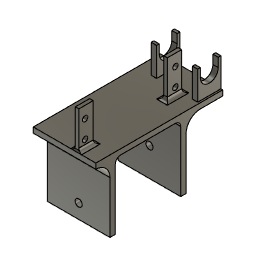
Servo_bracket v13 (Autodesk Fusion 360 design; units mm, degrees)
Autodesk Fusion 360 part; units mm, degrees
sketch "Sketch1" plane through (0, 0, 0) normal (0, 0, 1) x (1, 0, 0)
  line L0 (0, 0) -> (35, 0)
  line L1 (35, 0) -> (35, 71)
  line L2 (35, 71) -> (0, 71)
  line L3 (0, 71) -> (0, 0)
  dimension "d1" = 35
  dimension "d2" = 71
  constraint horizontal L0
  constraint vertical L1
  constraint horizontal L2
  constraint vertical L3
  constraint coincident L0.start L3.end
  measures "d1" distance of L0.start L0.end
  measures "d2" distance of L0.start L2.end
extrude "Extrude1" add sketch "Sketch1" along normal blind 3
sketch "Sketch2" plane through (0, 0, 3) normal (0, 0, 1) x (-1, 0, 0)
  line L0 (0, -71) -> (0, 0)
  line L1 (0, 0) -> (-35, 0)
  line L2 (-35, 0) -> (-35, -71)
  line L3 (-35, -71) -> (0, -71)
  line L4 (-25, -0.5) -> (-23, -0.5)
  line L5 (-23, -0.5) -> (-23, -8.5)
  line L6 (-23, -8.5) -> (-25, -8.5)
  line L7 (-25, -8.5) -> (-25, -0.5)
  line L8 (0, 0) -> (-35, 0)
  line L9 (-25, -58) -> (-23, -58)
  line L10 (-23, -58) -> (-23, -50)
  line L11 (-23, -50) -> (-25, -50)
  line L12 (-25, -50) -> (-25, -58)
  line L13 (-35, 0) -> (-35, -71)
  dimension "d5" = 0.5
  dimension "d6" = 2
  dimension "d7" = 8
  dimension "d8" = 2
  dimension "d9" = 8
  dimension "d10" = 41.5
  dimension "d11" = 10
  dimension "d12" = 10
  constraint horizontal L4
  constraint vertical L5
  constraint horizontal L6
  constraint vertical L7
  constraint horizontal L9
  constraint vertical L10
  constraint horizontal L11
  constraint vertical L12
  measures "d5" distance of L4 L8
  measures "d6" distance of L5.end L6.end
  measures "d7" distance of L4.end L5.end
  measures "d8" distance of L9.start L9.end
  measures "d9" distance of L9.end L10.end
  measures "d10" distance of L6 L11
  measures "d11" distance of L7 L13
  measures "d12" distance of L12 L13
extrude "Extrude2" add sketch "Sketch2" along normal blind 21 contours L4 L5 L6 L7 | L9 L10 L11 L12
sketch "Sketch4" plane through (25, 0, 0) normal (1, 0, 0) x (0, 1, 0)
  line L0 (0.5, 3) -> (8.5, 3)
  line L1 (8.5, 3) -> (8.5, 24)
  line L2 (8.5, 24) -> (0.5, 24)
  line L3 (0.5, 24) -> (0.5, 3)
  circle A0 centre (4, 7.5) radius 1.5
  circle A1 centre (4, 17.5) radius 1.5
  circle A2 centre (54.5, 7.5) radius 1.5
  circle A3 centre (54.5, 17.5) radius 1.5
  line L4 (58, 3) -> (50, 3)
  line L5 (50, 3) -> (50, 24)
  dimension "d15" = 3
  dimension "d16" = 4.5
  dimension "d17" = 3.5
  dimension "d18" = 3
  dimension "d19" = 10
  dimension "d20" = 3.5
  dimension "d21" = 3
  dimension "d22" = 3
  dimension "d23" = 4.5
  dimension "d24" = 4.5
  dimension "d25" = 10
  dimension "d26" = 4.5
  measures "d15" diameter of A0
  measures "d16" distance of L0 A0.centre
  measures "d17" distance of L3 A0.centre
  measures "d18" diameter of A1
  measures "d19" distance of A0.centre A1.centre
  measures "d20" distance of L3 A1.centre
  measures "d21" diameter of A2
  measures "d22" diameter of A3
  measures "d23" distance of A2.centre L4
  measures "d24" distance of A2.centre L5
  measures "d25" distance of A2.centre A3.centre
  measures "d26" distance of A3.centre L5
extrude "Extrude3" cut sketch "Sketch4" against normal up to surface (2 mm away) contours A0 | A1 | A2 | A3
sketch "Sketch5" plane through (0, 0, 3) normal (0, 0, 1) x (-1, 0, 0)
  line L0 (-25, -8.5) -> (-25, -0.5)
  line L1 (-25, -0.5) -> (-23, -0.5)
  line L2 (-23, -0.5) -> (-23, -8.5)
  line L3 (-23, -8.5) -> (-25, -8.5)
  line L4 (-25, -50) -> (-23, -50)
  line L5 (-23, -50) -> (-23, -58)
  line L6 (-23, -58) -> (-25, -58)
  line L7 (-25, -58) -> (-25, -50)
  line L8 (0, -71) -> (0, 0)
  line L9 (0, 0) -> (-35, 0)
  line L10 (-35, 0) -> (-35, -71)
  line L11 (-35, -71) -> (0, -71)
  line L12 (-31, -58) -> (-34, -58)
  line L13 (-34, -58) -> (-34, -71)
  line L14 (-34, -71) -> (-31, -71)
  line L15 (-31, -71) -> (-31, -58)
  line L16 (-8, -58) -> (-11, -58)
  line L17 (-11, -58) -> (-11, -71)
  line L18 (-11, -71) -> (-8, -71)
  line L19 (-8, -71) -> (-8, -58)
  dimension "d30" = 13
  dimension "d31" = 3
  dimension "d32" = 1
  dimension "d33" = 13
  dimension "d34" = 3
  dimension "d37" = 20
  constraint horizontal L12
  constraint vertical L13
  constraint horizontal L14
  constraint vertical L15
  constraint horizontal L16
  constraint vertical L17
  constraint horizontal L18
  constraint vertical L19
  constraint coincident L10.end L14
  constraint coincident L8.start L18
  measures "d30" distance of L12.start L14.end
  measures "d31" distance of L12.start L12.end
  measures "d32" distance of L10 L13
  measures "d33" distance of L16.start L18.end
  measures "d34" distance of L16.start L16.end
  measures "d37" distance of L15 L17
extrude "Extrude4" add sketch "Sketch5" along normal blind 16 contours L11 L16 L17 L18 L19 | L11 L12 L13 L14 L15
sketch "Sketch6" plane through (34, 0, 0) normal (1, 0, 0) x (0, 1, 0)
  line L0 (58, 3) -> (71, 3)
  line L1 (71, 3) -> (71, 19)
  line L2 (71, 19) -> (58, 19)
  line L3 (58, 19) -> (58, 3)
  line L4 (59.5, 14) -> (59.5, 19)
  line L5 (69.5, 14) -> (69.5, 19)
  line L6 (59.5, 19) -> (69.5, 19)
  arc A0 (59.5, 14) -> (69.5, 14) centre (64.5, 14) ccw
  dimension "d40" = 10
  dimension "d42" = 1.5
  dimension "d43" = 11
  constraint coincident L2 L4.end
  constraint tangent L4 A0
  constraint perpendicular L2 L4
  constraint coincident L2 L5.end
  constraint tangent L5 A0
  constraint perpendicular L2 L5
  measures "d40" diameter of A0
  measures "d42" distance of L3 L4
  measures "d43" distance of L0 A0.centre
extrude "Extrude8" cut sketch "Sketch6" against normal up to surface (26 mm away) contours L2 L4 L5 L6 A0
extrude "Extrude5" cut sketch "Sketch6" against normal up to surface (26 mm away) contours L2 L4 L5 L6 A0
fillet "Fillet1" radius 2 3 edges at (25, 4.5, 3) (24, 8.5, 3) (23, 4.5, 3)
fillet "Fillet2" radius 1 1 edges at (24, 0.5, 3)
fillet "Fillet3" radius 2 4 edges at (25, 54, 3) (24, 50, 3) (23, 54, 3) (24, 58, 3)
sketch "Sketch8" plane through (0, 0, 3) normal (0, 0, 1) x (-1, 0, 0)
  line L0 (-31, -71) -> (-11, -71)
  line L1 (-34, -71) -> (-34, -58)
  line L2 (-34, -58) -> (-31, -58)
  line L3 (-31, -58) -> (-31, -71)
  line L4 (-8, -71) -> (0, -71)
  line L5 (-11, -71) -> (-11, -58)
  line L6 (-11, -58) -> (-8, -58)
  line L7 (-8, -58) -> (-8, -71)
  line L8 (-21, 0) -> (-21, -10.5)
  line L9 (-21, -10.5) -> (-27, -10.5)
  line L10 (-27, -10.5) -> (-27, 0)
  line L11 (-27, 0) -> (-35, 0)
  line L12 (-35, 0) -> (-35, -71)
  line L13 (-35, -71) -> (-34, -71)
  line L14 (0, -71) -> (0, 0)
  line L15 (0, 0) -> (-21, 0)
  line L16 (-21, -60) -> (-27, -60)
  line L17 (-27, -60) -> (-27, -48)
  line L18 (-27, -48) -> (-21, -48)
  line L19 (-21, -48) -> (-21, -60)
  line L20 (-12, -21.25) -> (-26, -21.25)
  line L21 (-26, -21.25) -> (-26, -30)
  line L22 (-26, -30) -> (-12, -30)
  line L23 (-12, -30) -> (-12, -21.25)
  dimension "d60" = 14
  dimension "d61" = 8.75
  dimension "d62" = 12
  dimension "d63" = 21.25
  constraint horizontal L20
  constraint vertical L21
  constraint horizontal L22
  constraint vertical L23
  measures "d60" distance of L21.end L22.end
  measures "d61" distance of L20.start L22.end
  measures "d62" distance of L14 L23
  measures "d63" distance of L11 L20
sketch "Sketch9" plane through (0, 0, 0) normal (0, 0, -1) x (1, 0, 0)
  line L0 (0, 0) -> (0, -71)
  line L1 (0, -71) -> (35, -71)
  line L2 (35, -71) -> (35, 0)
  line L3 (35, 0) -> (0, 0)
  line L4 (35, -7.9) -> (0, -7.9)
  line L5 (0, -7.9) -> (0, -10.9)
  line L6 (0, -10.9) -> (35, -10.9)
  line L7 (35, -10.9) -> (35, -7.9)
  line L8 (35, -47.5) -> (0, -47.5)
  line L9 (0, -47.5) -> (0, -50.5)
  line L10 (0, -50.5) -> (35, -50.5)
  line L11 (35, -50.5) -> (35, -47.5)
  dimension "d70" = 10.9
  dimension "d71" = 23.5
  dimension "d72" = 3
  dimension "d73" = 3
  constraint horizontal L4
  constraint vertical L5
  constraint horizontal L6
  constraint vertical L7
  constraint coincident L0 L5.end
  constraint coincident L2 L4.start
  constraint horizontal L8
  constraint vertical L9
  constraint horizontal L10
  constraint vertical L11
  constraint coincident L0 L9.end
  constraint coincident L2 L8.start
  measures "d70" distance of L3 L6
  measures "d71" distance of L1 L8
  measures "d72" distance of L8.start L10.end
  measures "d73" distance of L4.end L5.end
extrude "Extrude9" add sketch "Sketch9" along normal blind 37 contours L0 L2 L4 L5 L6 L7 | L0 L2 L8 L9 L10 L11
sketch "Sketch10" plane through (0, 50.5, 0) normal (0, 1, 0) x (-1, 0, 0)
  line L0 (-35, 0) -> (-35, -37)
  line L1 (-35, -37) -> (0, -37)
  line L2 (0, -37) -> (0, 0)
  circle A0 through (-15.5, -29, -42.6) (-18.5, -27.2679, -42.6) (-18.5, -30.7321, -42.6)
  line L3 (-35, 0, -42.6) -> (-35, -37, -42.6)
  line L4 (-35, -37, -42.6) -> (0, -37, -42.6)
  line L5 (0, 0) -> (-35, 0)
  dimension "d82" = 4
  dimension "d83" = 17.5
  dimension "d84" = 8
sketch "Sketch11" plane through (0, 50.5, 0) normal (0, 1, 0) x (-1, 0, 0)
  circle A0 centre (-17.5, -21) radius 2
  line L0 (0, -37) -> (0, 0)
  line L1 (-35, -37) -> (0, -37)
  dimension "d79" = 4
  dimension "d80" = 17.5
  dimension "d81" = 16
  measures "d79" diameter of A0
  measures "d80" distance of A0.centre L0
  measures "d81" distance of A0.centre L1
extrude "Extrude10" cut sketch "Sketch10" along normal up to surface (3 mm away) contours A0 in plane through (0, 7.9, 0) normal (0, 1, 0)
extrude "Extrude11" cut sketch "Sketch11" against normal up to surface (3 mm away)
fillet "Fillet6" radius 8 2 edges at (17.5, 7.9, 0) (17.5, 50.5, 0)
fillet "Fillet7" radius 3 2 edges at (17.5, 10.9, 0) (17.5, 47.5, 0)
